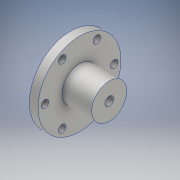
# Autodesk Inventor part: 10mmkethub18025
Saved by Autodesk Inventor 2019 (Build 230136000, 136)
## iProperties
Created: 2018-09-03
Part Number: 10mmkethub18025
Material: 一般
Document SubType Name: Modeling
Designer: シュンダイ
Density: 1 g/cm^3
Appearance: アルミニウム - フラット
Author: シュンダイ
Autodesk Inventor part; units mm, degrees
ref_plane "YZ Plane" through (0, 0, 0) normal (1, 0, 0) x (0, 1, 0)
ref_plane "XZ Plane" through (0, 0, 0) normal (0, 1, 0) x (-1, 0, 0)
ref_plane "XY Plane" through (0, 0, 0) normal (0, 0, 1) x (1, 0, 0)
sketch "スケッチ1" plane through (0, 0, 0) normal (1, 0, 0) x (0, 1, 0)
  point P0 (0, 0)
sketch "スケッチ2" plane through (0, 0, 0) normal (1, 0, 0) x (0, 1, 0)
  circle A0 centre (0, 0) radius 28.4
  dimension "d0" = 56.8
  constraints: 1 centre point, 1 coincident
  measures "d0" diameter of A0
extrude "押し出し1" add sketch "スケッチ2" along normal blind 6
sketch "スケッチ3" plane through (6, 0, 0) normal (1, 0, 0) x (0, 0, -1)
  circle A0 centre (0, 0) radius 12
  dimension "d3" = 24
  constraints: 1 centre point, 1 coincident
  measures "d3" diameter of A0
extrude "押し出し2" add sketch "スケッチ3" along normal blind 20.4
sketch "スケッチ8" plane through (26.4, 0, 0) normal (1, 0, 0) x (0, 0, -1)
  circle A0 centre (0, 0) radius 12 projected
  constraints: 1 coincident
hole "穴2" at (26.4, 0, 0) direction (-1, 0, 0) diameter 6 end through all
sketch "スケッチ7" plane through (0, 0, 0) normal (-1, 0, 0) x (0, 0, 1)
  circle A0 centre (0, 0) radius 23.75
  line L0 (0, -23.75) -> (-20.5681, -11.875)
  line L1 (-20.5681, -11.875) -> (-20.5681, 11.875)
  line L2 (-20.5681, 11.875) -> (0, 23.75)
  line L3 (0, 23.75) -> (20.5681, 11.875)
  line L4 (20.5681, 11.875) -> (20.5681, -11.875)
  line L5 (20.5681, -11.875) -> (0, -23.75)
  dimension "d43" = 47.5
  constraints: 12 end point, 2 coincident, 1 vertical alignment, 15 other
hole "穴3" at (0, 11.875, 20.5681) at (0, 23.75, 0) at (0, -11.875, 20.5681) at (0, -23.75, 0) at (0, -11.875, -20.5681) at (0, 11.875, -20.5681) direction (1, 0, 0) diameter 5.2 end through all
